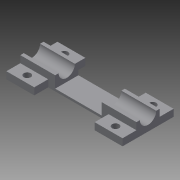
# Autodesk Inventor part: bearing bed
Saved by Autodesk Inventor 2013 SP2 (Build 170200200, 200)
## iProperties
Created: 2017-05-18
Part Number: bearing bed
Material: Generic
Document SubType Name: Modeling
Designer: Herman de Vries
Density: 1 g/cm^3
Author: Herman de Vries
Autodesk Inventor part; units mm, degrees
ref_plane "YZ Plane" through (0, 0, 0) normal (1, 0, 0) x (0, 1, 0)
ref_plane "XZ Plane" through (0, 0, 0) normal (0, 1, 0) x (-1, 0, 0)
ref_plane "XY Plane" through (0, 0, 0) normal (0, 0, 1) x (1, 0, 0)
sketch "Sketch1" plane through (0, 0, 0) normal (0, 0, 1) x (1, 0, 0)
  line L0 (0, 0) -> (50, 0)
  line L1 (50, 0) -> (50, 10)
  line L2 (50, 10) -> (0, 10)
  line L3 (0, 10) -> (0, 0)
  dimension "d0" = 50
  dimension "d1" = 10
  constraints: 8 end point, 2 parallel, 1 horizontal, 1 perpendicular
  measures "d0" distance of L2.end L1.end
  measures "d1" distance of L2.end L0.start
extrude "Extrusion1" add sketch "Sketch1" along normal blind 6
sketch "Sketch2" plane through (0, 0, 0) normal (-1, 0, 0) x (0, 0, 1)
  circle A0 centre (6, 5) radius 3.5
  line L0 (6, 10) -> (6, 0) projected
  point P0 (0, 0)
  dimension "d4" = 7
  constraints: 1 centre point, 1 coincident, 1 midpoint
  measures "d4" diameter of A0
extrude "Extrusion2" cut sketch "Sketch2" against normal through all
sketch "Sketch3" plane through (0, 0, 0) normal (0, 0, -1) x (-1, 0, 0)
  line L0 (-50, 0) -> (-50, 10) projected
  line L1 (0, 10) -> (0, 0) projected
  line L2 (-50, 10) -> (-38, 10)
  line L3 (-38, 10) -> (-38, 16)
  line L4 (-38, 16) -> (-50, 16)
  line L5 (-50, 16) -> (-50, 10)
  line L6 (0, 10) -> (-12, 10)
  line L7 (-12, 10) -> (-12, 16)
  line L8 (-12, 16) -> (0, 16)
  line L9 (0, 16) -> (0, 10)
  line L10 (0, 0) -> (-12, 0)
  line L11 (-12, 0) -> (-12, -6)
  line L12 (-12, -6) -> (0, -6)
  line L13 (0, -6) -> (0, 0)
  line L14 (-50, 0) -> (-38, 0)
  line L15 (-38, 0) -> (-38, -6)
  line L16 (-38, -6) -> (-50, -6)
  line L17 (-50, -6) -> (-50, 0)
  circle A0 centre (-44, 13) radius 1.5
  circle A1 centre (-6, 13) radius 1.5
  circle A2 centre (-6, -3) radius 1.5
  circle A3 centre (-44, -3) radius 1.5
  point P0 (-38, 13)
  point P1 (-12, 13)
  point P2 (-12, -3)
  point P3 (-50, -3)
  point P4 (-44, 16)
  point P5 (-6, 16)
  point P6 (-6, 0)
  point P7 (-44, 0)
  dimension "d15" = 12
  dimension "d16" = 6
  dimension "d17" = 12
  dimension "d18" = 6
  dimension "d19" = 12
  dimension "d20" = 6
  dimension "d21" = 12
  dimension "d22" = 6
  dimension "d23" = 3
  dimension "d24" = 3
  dimension "d25" = 3
  dimension "d26" = 3
  constraints: 32 end point, 8 midpoint, 8 parallel, 4 centre point, 4 horizontal, 4 horizontal alignment, 4 perpendicular, 4 vertical alignment
  measures "d15" distance of L4.end L3.end
  measures "d16" distance of L3.end L2.end
  measures "d17" distance of L7.end L8.end
  measures "d18" distance of L6.end L7.end
  measures "d19" distance of L12.end L11.end
  measures "d20" distance of L11.end L10.end
  measures "d21" distance of L15.end L16.end
  measures "d22" distance of L14.end L15.end
  measures "d23" diameter of A0
  measures "d24" diameter of A1
  measures "d25" diameter of A2
  measures "d26" diameter of A3
extrude "Extrusion3" add sketch "Sketch3" against normal blind 3
sketch "Sketch4" plane through (0, 0, 6) normal (0, 0, 1) x (1, 0, 0)
  line L0 (50, 10) -> (0, 10) projected
  line L1 (0, 0) -> (50, 0) projected
  line L2 (15, 10) -> (35, 10)
  line L3 (35, 10) -> (35, 0)
  line L4 (35, 0) -> (15, 0)
  line L5 (15, 0) -> (15, 10)
  point P0 (25, 10)
  dimension "d29" = 20
  constraints: 8 end point, 2 midpoint, 2 parallel, 2 point on line, 1 horizontal, 1 perpendicular
  measures "d29" distance of L2.start L2.end
extrude "Extrusion4" cut sketch "Sketch4" against normal blind 5
equation "\"d15\" = d21"
equation "\"d17\" = d21"
equation "\"d19\" = d21"
body "Solid1"
